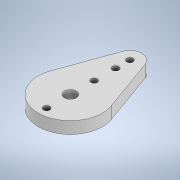
# Autodesk Inventor part: Beam support
Saved by Autodesk Inventor 2022 (Build 260153000, 153)
## iProperties
Created: 2022-03-02
Part Number: Beam support
Material: Genérico
Document SubType Name: Modeling
Designer: JK
Density: 1 g/cm^3
Appearance: Valor por defecto
Author: JK
Autodesk Inventor part; units mm, degrees
ref_plane "YZ Plane" through (0, 0, 0) normal (1, 0, 0) x (0, 1, 0)
ref_plane "XZ Plane" through (0, 0, 0) normal (0, 1, 0) x (-1, 0, 0)
ref_plane "XY Plane" through (0, 0, 0) normal (0, 0, 1) x (1, 0, 0)
sketch "Boceto1" plane through (0, 0, 0) normal (0, 1, 0) x (-1, 0, 0)
  circle A0 centre (0, 0) radius 27
  circle A1 centre (0, -50) radius 10
  circle A2 centre (0, 0) radius 5
  line L0 (25.3915, -9.18) -> (9.4043, -53.4)
  line L1 (-25.3915, -9.18) -> (-9.4043, -53.4)
  circle A3 centre (0, -50) radius 2.7
  circle A4 centre (0, -38) radius 2.7
  circle A5 centre (0, -20) radius 2.7
  circle A6 centre (0, 20) radius 2.7
  dimension "d0" = 10
  dimension "d1" = 5.4
  dimension "d2" = 5.4
  dimension "d3" = 12
  dimension "d4" = 50
  dimension "d5" = 20
  dimension "d6" = 54
  dimension "d10" = 5.4
  dimension "d11" = 5.4
  dimension "d12" = 20
  dimension "d13" = 20
  constraints: 7 centre point, 4 end point, 4 point on circle, 4 tangent, 3 coincident, 1 vertical alignment
  measures "d0" diameter of A2
  measures "d1" diameter of A4
  measures "d2" diameter of A3
  measures "d3" distance of A4.centre A1.centre
  measures "d4" distance of A1.centre point (0, 0)
  measures "d5" diameter of A1
  measures "d6" diameter of A0
  measures "d10" diameter of A6
  measures "d11" diameter of A5
  measures "d12" distance of A5.centre point (0, 0)
  measures "d13" distance of point (0, 0) A6.centre
extrude "Extrusión1" add sketch "Boceto1" along normal blind 10 contours A0 | A0 L0 A1 A4 L1 | A1 A4 picked at (1.999, -42.9031)
